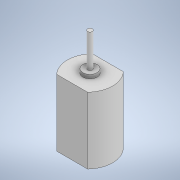
# Autodesk Inventor part: FläktMotor
Saved by Autodesk Inventor 2021 (Build 250183000, 183)
## iProperties
Created: 2025-01-14
Part Number: FläktMotor
Material: Generic
Document SubType Name: Modeling
Designer: 24lucsil
Density: 1 g/cm^3
Appearance: Default
Author: 24lucsil
Autodesk Inventor part; units mm, degrees
ref_plane "YZ Plane" through (0, 0, 0) normal (1, 0, 0) x (0, 1, 0)
ref_plane "XZ Plane" through (0, 0, 0) normal (0, 1, 0) x (-1, 0, 0)
ref_plane "XY Plane" through (0, 0, 0) normal (0, 0, 1) x (1, 0, 0)
sketch "Sketch1" plane through (0, 0, 0) normal (0, 1, 0) x (-1, 0, 0)
  line L0 (0, 0) -> (-6.5, 0)
  line L1 (0, 0) -> (6.5, 0)
  line L2 (6.5, 0) -> (6.5, -15) construction
  line L3 (6.5, -15) -> (-6.5, -15)
  line L4 (-6.5, 0) -> (-9.5, 0) construction
  line L5 (6.5, 0) -> (9.5, 0) construction
  arc A0 (-6.5, 0) -> (-6.5, -15) centre (1.375, -7.5) ccw
  arc A1 (6.5, -15) -> (6.5, 0) centre (-1.375, -7.5) ccw
  dimension "d0" = 6.5
  dimension "d1" = 6.5
  dimension "d2" = 15
  dimension "d3" = 13
  dimension "d4" = 3
  dimension "d5" = 3
  constraints: 12 end point, 5 horizontal, 4 point on circle, 2 centre point, 1 vertical
  measures "d0" distance of L0.start L1.end
  measures "d1" distance of L0.start L0.end
  measures "d2" distance of L1.end L2.end
  measures "d3" distance of L2.end L3.end
  measures "d4" distance of L0.end L4.end
  measures "d5" distance of L1.end L5.end
extrude "Extrusion1" add sketch "Sketch1" along normal blind 28
sketch "Sketch2" plane through (0, 28, 0) normal (0, 1, 0) x (1, 0, 0)
  line L0 (0, 0) -> (0, 7.5) construction
  circle A0 centre (0, 7.5) radius 3
  dimension "d8" = 7.5
  dimension "d9" = 6
  constraints: 2 end point, 1 centre point, 1 coincident, 1 vertical
  measures "d8" distance of L0.start L0.end
  measures "d9" diameter of A0
extrude "Extrusion2" add sketch "Sketch2" along normal blind 1.6
sketch "Sketch3" plane through (0, 29.6, -7.5) normal (0, 1, 0) x (1, 0, 0)
  circle A0 centre (0, 0) radius 1
  point P0 (0, -7.5)
  dimension "d12" = 2
  constraints: 1 centre point
  measures "d12" diameter of A0
extrude "Extrusion3" add sketch "Sketch3" along normal blind 14
body "Solid1"
